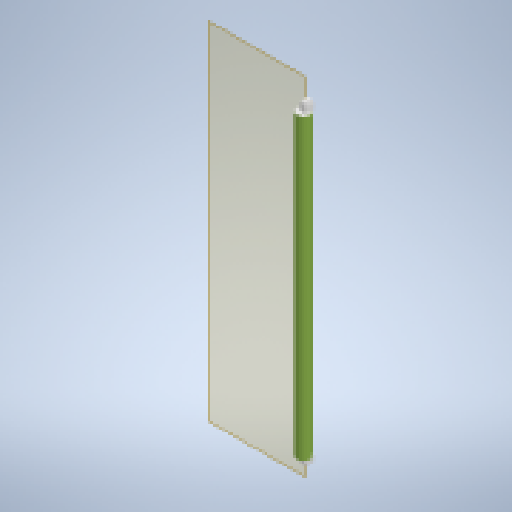
# Autodesk Inventor part: canvas-cover-stowed
Saved by Autodesk Inventor 2023 (Build 270158030, 158C)
## iProperties
Created: 2024-09-25
Part Number: canvas-cover-stowed
Material: Generic
Document SubType Name: Modeling
Designer: Imogen Heard
Density: 1 g/cm^3
Appearance: Default
Author: Imogen Heard
Autodesk Inventor part; units mm, degrees
ref_plane "YZ Plane" through (0, 0, 0) normal (1, 0, 0) x (0, 1, 0)
ref_plane "XZ Plane" through (0, 0, 0) normal (0, 1, 0) x (-1, 0, 0)
ref_plane "XY Plane" through (0, 0, 0) normal (0, 0, 1) x (1, 0, 0)
ref_plane "Work Plane1" through (0, 0, 0) normal (0, 0, 1) x (1, 0, 0)
sketch "Sketch1" plane through (0, 0, 0) normal (0, 0, 1) x (1, 0, 0)
  line L0 (0, 0) -> (700, 0) projected
  line L1 (700, 0) -> (700, 1930) projected
  line L2 (0, 1930) -> (700, 1930) projected
  line L3 (0, 0) -> (0, 1930) projected
  line L4 (700, 0) -> (650, 0)
  line L5 (650, 0) -> (650, 50)
  line L6 (650, 50) -> (700, 50)
  line L7 (700, 50) -> (700, 0)
  line L8 (700, 1930) -> (650, 1930)
  line L9 (650, 1930) -> (650, 1880)
  line L10 (650, 1880) -> (700, 1880)
  line L11 (700, 1880) -> (700, 1930)
  dimension "d0" = 50
  dimension "d1" = 50
  dimension "d2" = 50
  dimension "d3" = 50
  constraints: 16 end point, 4 parallel, 2 horizontal, 2 perpendicular
  measures "d0" distance between parallel lines of L6 L0
  measures "d1" distance between parallel lines of L1 L5
  measures "d2" distance between parallel lines of L1 L9
  measures "d3" distance between parallel lines of L2 L10
extrude "Extrusion1" add sketch "Sketch1" along normal blind 50 contours L5 L6 L1 L0 | L2 L1 L10 L9
fillet "Fillet1" radius 20 10 edges at (675, 0, 50) (650, 25, 50) (700, 25, 50) (700, 0, 25) (650, 0, 25) (650, 1905, 50) (700, 1905, 50) (675, 1930, 50) (700, 1930, 25) (650, 1930, 25)
sketch "Sketch2" plane through (650, 50, 0) normal (0, 1, 0) x (1, 0, 0)
  circle A0 centre (25, -40) radius 40
  arc A1 (30, -50) -> (50, -30) centre (30, -30) ccw projected
  line L0 (50, 0) -> (50, -30) projected
  line L1 (50, 0) -> (0, 0) projected
  line L2 (0, 0) -> (0, -30) projected
  arc A2 (0, -30) -> (20, -50) centre (20, -30) ccw projected
  line L3 (30, -50) -> (20, -50) projected
  line L4 (-22.934, -16.6175) -> (-13.936, -55.5923) projected
  point P0 (-650, 0)
  dimension "d7" = 25
  dimension "d8" = 80
  dimension "d9" = 40
  constraints: 1 centre point
  measures "d7" distance from line of L0 A0.centre
  measures "d8" diameter of A0
  measures "d9" distance from line of L1 A0.centre
extrude "Extrusion2" add sketch "Sketch2" along normal up to surface (1830 mm away) separate body contours A0 L2 A2 L3 A1 L0 | L0 A1 L3 A2 L2 A0
body "Solid1"
body "Solid2"
